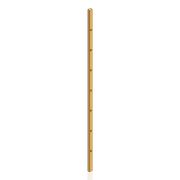
# Autodesk Inventor part: pieza
Saved by Autodesk Inventor 2020 (Build 240168000, 168)
## iProperties
Created: 2022-05-05
Part Number: pieza
Material: Generic
Document SubType Name: Modeling
Designer: leo
Density: 1 g/cm^3
Appearance: Yellow Pine - Solid Stained Light Low Gloss
Author: leo
Autodesk Inventor part; units mm, degrees
ref_plane "YZ Plane" through (0, 0, 0) normal (1, 0, 0) x (0, 1, 0)
ref_plane "XZ Plane" through (0, 0, 0) normal (0, 1, 0) x (-1, 0, 0)
ref_plane "XY Plane" through (0, 0, 0) normal (0, 0, 1) x (1, 0, 0)
sketch "Sketch1" plane through (0, 0, 0) normal (0, 1, 0) x (-1, 0, 0)
  line L0 (15, 20) -> (-15, 20)
  line L1 (-15, 20) -> (-15, -20)
  line L2 (-15, -20) -> (15, -20)
  line L3 (15, -20) -> (15, 20)
  point P0 (0, 0)
  point P1 (15, 0)
  point P2 (0, -20)
  dimension "d0" = 40
  dimension "d1" = 30
  constraints: 8 end point, 2 midpoint, 2 parallel, 1 horizontal, 1 horizontal alignment, 1 perpendicular, 1 vertical alignment
  measures "d0" distance of L2.end L0.start
  measures "d1" distance of L1.end L2.end
extrude "Extrusion1" add sketch "Sketch1" along normal mid plane 2400
sketch "Sketch2" plane through (0, 0, 0) normal (0, 0, 1) x (1, 0, 0)
  line L0 (35, 0) -> (-35, 0)
  line L1 (-35, 0) -> (-35, -12.5)
  line L2 (-35, -12.5) -> (-10, -12.5)
  line L3 (-10, -12.5) -> (-10, -5)
  line L4 (-10, -5) -> (10, -5)
  line L5 (10, -5) -> (10, -12.5)
  line L6 (10, -12.5) -> (35, -12.5)
  line L7 (35, -12.5) -> (35, 0)
  point P0 (0, 0)
  point P1 (0, 0)
  dimension "d4" = 10
  dimension "d5" = 70
  dimension "d6" = 25
  dimension "d7" = 20
  constraints: 16 end point, 7 perpendicular, 2 equal length, 1 coincident, 1 horizontal, 1 midpoint
  measures "d4" diameter of L4 L0
  measures "d5" distance of L0.start L0.end
  measures "d6" diameter of L6 L0
  measures "d7" distance between parallel lines of L3 L5
revolve "Revolution1" cut sketch "Sketch2" angle 360 about axis through (35, 0, 0) along (-1, 0, 0)
pattern_linear "Rectangular Pattern1" count 7 spacing 300 along (0, 1, 0) of "Revolution1" first direction both ways yes
body "Solid1"
